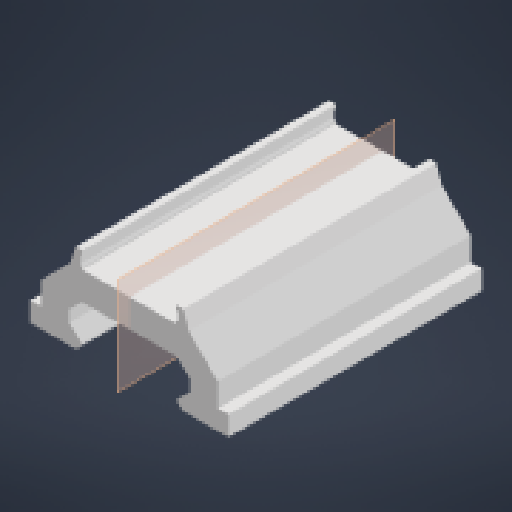
# Autodesk Inventor part: Rail clamp
Saved by Autodesk Inventor 2023 (Build 270158000, 158)
## iProperties
Created: 2023-10-16
Part Number: Rail clamp
Material: Generic
Document SubType Name: Modeling
Designer: nick_
Density: 1 g/cm^3
Appearance: Default
Author: nick_
Autodesk Inventor part; units mm, degrees
ref_plane "YZ Plane" through (0, 0, 0) normal (1, 0, 0) x (0, 1, 0)
ref_plane "XZ Plane" through (0, 0, 0) normal (0, 1, 0) x (-1, 0, 0)
ref_plane "XY Plane" through (0, 0, 0) normal (0, 0, 1) x (1, 0, 0)
sketch "Sketch1" plane through (0, 0, 0) normal (0, 0, 1) x (1, 0, 0)
  line L0 (6.1935, -6.1609) -> (-18.8065, -6.1609) construction
  line L1 (6.1935, -3.1609) -> (6.1935, -6.1609) construction
  line L2 (2.0882, -3.1609) -> (6.1935, -3.1609) construction
  line L3 (2.0882, -0.2145) -> (2.0882, -3.1609) construction
  line L4 (4.298, 1.9953) -> (2.0882, -0.2145) construction
  line L5 (4.298, 3.9511) -> (4.298, 1.9953) construction
  line L6 (2.0882, 6.1609) -> (4.298, 3.9511) construction
  line L7 (2.0882, 6.1609) -> (-14.7012, 6.1609) construction
  line L8 (-14.7012, 6.1609) -> (-16.911, 3.9511) construction
  line L9 (-16.911, 3.9511) -> (-16.911, 1.9953) construction
  line L10 (-16.911, 1.9953) -> (-14.7012, -0.2145) construction
  line L11 (-14.7012, -0.2145) -> (-14.7012, -3.1609) construction
  line L12 (-14.7012, -3.1609) -> (-18.8065, -3.1609) construction
  line L13 (-18.8065, -3.1609) -> (-18.8065, -6.1609) construction
  line L14 (2.1882, -3.0609) -> (6.2935, -3.0609)
  line L15 (6.2935, -3.0609) -> (6.2935, -6.2609)
  line L16 (6.2935, -6.2609) -> (-18.9065, -6.2609)
  line L17 (-18.9065, -6.2609) -> (-18.9065, -3.0609)
  line L18 (-18.9065, -3.0609) -> (-14.8012, -3.0609)
  line L19 (-14.8012, -3.0609) -> (-14.8012, -0.2559)
  line L20 (-14.8012, -0.2559) -> (-17.011, 1.9539)
  line L21 (-17.011, 1.9539) -> (-17.011, 3.9925)
  line L22 (-17.011, 3.9925) -> (-14.7427, 6.2609)
  line L23 (-14.7427, 6.2609) -> (2.1296, 6.2609)
  line L24 (2.1296, 6.2609) -> (4.398, 3.9925)
  line L25 (4.398, 3.9925) -> (4.398, 1.9539)
  line L26 (4.398, 1.9539) -> (2.1882, -0.2559)
  line L27 (2.1882, -0.2559) -> (2.1882, -3.0609)
  line L28 (11.2935, 1.9391) -> (9.398, 1.9391)
  line L29 (9.398, 1.9391) -> (9.398, 6.0636)
  line L30 (9.398, 6.0636) -> (4.2007, 11.2609)
  line L31 (4.2007, 11.2609) -> (-16.8137, 11.2609)
  line L32 (-16.8137, 11.2609) -> (-22.011, 6.0636)
  line L33 (-22.011, 6.0636) -> (-22.011, 1.9391)
  line L34 (-22.011, 1.9391) -> (-23.9065, 1.9391)
  line L35 (-23.9065, 1.9391) -> (-23.9065, -1.5609)
  line L36 (11.2935, -1.5609) -> (11.2935, 1.9391)
  line L37 (2.1882, -1.5609) -> (11.2935, -1.5609)
  line L38 (-14.8012, -1.5609) -> (-23.9065, -1.5609)
  point P0 (0, 0)
  point P1 (6.7408, -1.5609)
  point P2 (-19.3539, -1.5609)
  dimension "d0" = 0.1
  dimension "d1" = 5
  dimension "d2" = 1.5
  dimension "d3" = 5
  dimension "d5" = 5
  constraints: 50 end point, 2 midpoint, 2 perpendicular, 2 point on line, 1 horizontal alignment, 19 other
  measures "d0" distance between parallel lines of L3 L27
  measures "d1" distance between parallel lines of L36 L15
  measures "d2" distance between parallel lines of L37 L14
  measures "d3" distance between parallel lines of L31 L23
  measures "d5" distance between parallel lines of L35 L17
extrude "Extrusion1" add sketch "Sketch1" against normal blind 45 contours L27 L26 L25 L24 L23 L22 L21 L20 L19 L38 L35 L34 L33 L32 L31 L30 L29 L28 L36 L37
chamfer "Chamfer1" distance 1 angle 45 2 edges at (-14.8012, -1.5609, -22.5) (2.1882, -1.5609, -22.5)
sketch "Sketch3" plane through (0, 0, -45) normal (0, 0, -1) x (-1, 0, 0)
  line L0 (-2.2533, 11.7609) -> (14.8667, 11.7609) construction
  line L1 (14.8667, 11.7609) -> (14.8667, 13.2909) construction
  line L2 (-2.2533, 13.2909) -> (14.8667, 13.2909) construction
  line L3 (-2.2533, 11.7609) -> (-2.2533, 13.2909) construction
  line L4 (-2.1882, -0.5609) -> (-3.1882, -1.5609) construction
  line L5 (-2.1882, -0.5609) -> (-2.1882, -0.2559) construction
  line L6 (-2.1882, -0.2559) -> (-4.398, 1.9539) construction
  line L7 (-4.398, 1.9539) -> (-4.398, 3.9925) construction
  line L8 (-4.398, 3.9925) -> (-2.1296, 6.2609) construction
  line L9 (-2.1296, 6.2609) -> (14.7427, 6.2609) construction
  line L10 (14.7427, 6.2609) -> (17.011, 3.9925) construction
  line L11 (17.011, 3.9925) -> (17.011, 1.9539) construction
  line L12 (17.011, 1.9539) -> (14.8012, -0.2559) construction
  line L13 (14.8012, -0.2559) -> (14.8012, -0.5609) construction
  line L14 (15.8012, -1.5609) -> (14.8012, -0.5609) construction
  line L15 (15.8012, -1.5609) -> (23.9065, -1.5609) construction
  line L16 (23.9065, -1.5609) -> (23.9065, 1.9391) construction
  line L17 (23.9065, 1.9391) -> (22.011, 1.9391) construction
  line L18 (22.011, 1.9391) -> (22.011, 6.0636) construction
  line L19 (22.011, 6.0636) -> (16.8137, 11.2609) construction
  line L20 (16.8137, 11.2609) -> (-4.2007, 11.2609) construction
  line L21 (-4.2007, 11.2609) -> (-9.398, 6.0636) construction
  line L22 (-9.398, 6.0636) -> (-9.398, 1.9391) construction
  line L23 (-9.398, 1.9391) -> (-11.2935, 1.9391) construction
  line L24 (-11.2935, 1.9391) -> (-11.2935, -1.5609) construction
  line L25 (-11.2935, -1.5609) -> (-3.1882, -1.5609) construction
  line L26 (-2.0533, 11.2609) -> (-2.0533, 11.5609)
  line L27 (-2.0533, 11.5609) -> (-2.4533, 11.9609)
  line L28 (-2.4533, 11.9609) -> (-2.4533, 13.0909)
  line L29 (-2.4533, 13.0909) -> (-2.0533, 13.4909)
  line L30 (-2.0533, 13.4909) -> (-2.0533, 14.1683)
  line L31 (-2.0533, 14.1683) -> (-3.2638, 14.1683)
  line L32 (-3.2638, 14.1683) -> (-4.2007, 11.2609)
  line L33 (-4.2007, 11.2609) -> (-2.0533, 11.2609)
  line L34 (-2.2533, 13.2909) -> (-2.5848, 13.6224) construction
  line L35 (-2.2533, 13.2909) -> (-1.7845, 13.2909) construction
  point P0 (0, 0)
  point P1 (-2.2533, 13.2909)
  dimension "d15" = 0.2
  dimension "d16" = 135
  dimension "d17" = 0.2
  constraints: 20 end point, 4 point on line, 2 equal length, 2 midpoint, 2 perpendicular, 1 collinear, 1 horizontal, 1 parallel, 1 vertical
  measures "d15" distance between parallel lines of L3 L28
  measures "d16" angle of L35 L34
  measures "d17" distance from line of L2.start L30
extrude "Extrusion3" add sketch "Sketch3" against normal up to surface (45 mm away)
ref_plane "Work Plane1" through (-6.3065, -1.5609, 0) normal (1, 0, 0) x (0, 0, -1)
mirror "Mirror1" about plane through (-6.3065, -1.5609, 0) normal (1, 0, 0) of "Extrusion3"
sketch "Sketch4" plane through (2.0533, 11.2609, 0) normal (0, 1, 0) x (1, 0, 0)
  line L0 (-8.4373, 26.9134) -> (-8.4438, 26.9134) construction
  line L1 (-8.4438, 26.9134) -> (-8.4438, 27.0673) construction
  spline S0 degree 2 poles (-8.4438, 27.0673) (-8.3053, 27.184) (-7.9925, 27.3177) (-7.7834, 27.3177) knots 0 0 0 1 2 2 2 construction
  spline S1 degree 2 poles (-7.7834, 27.3177) (-7.5759, 27.3177) (-7.2615, 27.1848) (-7.1229, 27.0673) knots 0 0 0 1 2 2 2 construction
  line L2 (-7.1229, 27.0673) -> (-7.1229, 26.9134) construction
  line L3 (-7.1229, 26.9134) -> (-7.1294, 26.9134) construction
  spline S2 degree 2 poles (-7.1294, 26.9134) (-7.1756, 26.9652) (-7.3109, 27.0698) (-7.392, 27.1087) knots 0 0 0 1 2 2 2 construction
  spline S3 degree 2 poles (-7.392, 27.1087) (-7.4787, 27.1508) (-7.6715, 27.1994) (-7.7834, 27.1994) knots 0 0 0 1 2 2 2 construction
  spline S4 degree 2 poles (-7.7834, 27.1994) (-7.8944, 27.1994) (-8.0913, 27.15) (-8.1748, 27.1087) knots 0 0 0 1 2 2 2 construction
  spline S5 degree 2 poles (-8.1748, 27.1087) (-8.2583, 27.0682) (-8.3912, 26.9644) (-8.4373, 26.9134) knots 0 0 0 1 2 2 2 construction
  line L4 (-9.0457, 18.8862) -> (-10.0457, 18.8862) construction
  line L5 (-10.0457, 18.8862) -> (-10.0457, 19.1374) construction
  spline S6 degree 2 poles (-10.0457, 19.1374) (-10.0457, 19.2266) (-10.0166, 19.3514) (-9.9833, 19.3992) knots 0 0 0 1 2 2 2 construction
  spline S7 degree 2 poles (-9.9833, 19.3992) (-9.9452, 19.4551) (-9.8277, 19.5183) (-9.7443, 19.5183) knots 0 0 0 1 2 2 2 construction
  spline S8 degree 2 poles (-9.7443, 19.5183) (-9.6794, 19.5183) (-9.5628, 19.4721) (-9.5222, 19.4308) knots 0 0 0 1 2 2 2 construction
  spline S9 degree 2 poles (-9.5222, 19.4308) (-9.4712, 19.3789) (-9.4185, 19.2387) (-9.4185, 19.1318) knots 0 0 0 1 2 2 2 construction
  line L6 (-9.4185, 19.1318) -> (-9.4185, 19.0191) construction
  line L7 (-9.4185, 19.0191) -> (-9.0457, 19.0191) construction
  line L8 (-9.0457, 19.0191) -> (-9.0457, 18.8862) construction
  spline S10 degree 2 poles (-9.8205, 17.6472) (-9.7499, 17.6472) (-9.6381, 17.5726) (-9.6065, 17.507) knots 0 0 0 1 2 2 2 construction
  line L9 (-9.6065, 17.507) -> (-9.6017, 17.507) construction
  spline S11 degree 2 poles (-9.6017, 17.507) (-9.5773, 17.5961) (-9.4485, 17.6942) (-9.3529, 17.6942) knots 0 0 0 1 2 2 2 construction
  spline S12 degree 2 poles (-9.3529, 17.6942) (-9.2783, 17.6942) (-9.164, 17.6374) (-9.1268, 17.5904) knots 0 0 0 1 2 2 2 construction
  spline S13 degree 2 poles (-9.1268, 17.5904) (-9.083, 17.5337) (-9.0457, 17.4049) (-9.0457, 17.3028) knots 0 0 0 1 2 2 2 construction
  line L10 (-9.0457, 17.3028) -> (-9.0457, 17.0159) construction
  line L11 (-9.0457, 17.0159) -> (-10.0457, 17.0159) construction
  line L12 (-10.0457, 17.0159) -> (-10.0457, 17.2809) construction
  spline S14 degree 2 poles (-10.0457, 17.2809) (-10.0457, 17.3878) (-10.032, 17.4948) (-10.0052, 17.5434) knots 0 0 0 1 2 2 2 construction
  spline S15 degree 2 poles (-10.0052, 17.5434) (-9.9769, 17.5977) (-9.8837, 17.6472) (-9.8205, 17.6472) knots 0 0 0 1 2 2 2 construction
  spline S16 degree 2 poles (-10.066, 19.9195) (-10.066, 20.084) (-9.8067, 20.2387) (-9.5457, 20.2387) knots 0 0 0 1 2 2 2 construction
  spline S17 degree 2 poles (-9.5457, 20.2387) (-9.2767, 20.2387) (-9.0247, 20.0823) (-9.0247, 19.9195) knots 0 0 0 1 2 2 2 construction
  spline S18 degree 2 poles (-9.0247, 19.9195) (-9.0247, 19.7541) (-9.2816, 19.5994) (-9.5449, 19.5994) knots 0 0 0 1 2 2 2 construction
  spline S19 degree 2 poles (-9.5449, 19.5994) (-9.8156, 19.5994) (-10.066, 19.7558) (-10.066, 19.9195) knots 0 0 0 1 2 2 2 construction
  line L13 (-10.0457, 17.8263) -> (-10.0457, 18.0078) construction
  line L14 (-10.0457, 18.0078) -> (-9.489, 18.2574) construction
  line L15 (-9.489, 18.2574) -> (-10.0457, 18.4989) construction
  line L16 (-10.0457, 18.4989) -> (-10.0457, 18.6836) construction
  line L17 (-10.0457, 18.6836) -> (-9.0457, 18.6836) construction
  line L18 (-9.0457, 18.6836) -> (-9.0457, 18.5507) construction
  line L19 (-9.0457, 18.5507) -> (-9.9072, 18.5507) construction
  line L20 (-9.9072, 18.5507) -> (-9.3213, 18.2898) construction
  line L21 (-9.3213, 18.2898) -> (-9.3213, 18.2088) construction
  line L22 (-9.3213, 18.2088) -> (-9.9072, 17.9502) construction
  line L23 (-9.9072, 17.9502) -> (-9.0457, 17.9502) construction
  line L24 (-9.0457, 17.9502) -> (-9.0457, 17.8263) construction
  line L25 (-9.0457, 17.8263) -> (-10.0457, 17.8263) construction
  spline S20 degree 2 poles (-10.0684, 20.669) (-10.0684, 20.8052) (-9.9258, 20.9697) (-9.814, 20.9697) knots 0 0 0 1 2 2 2 construction
  spline S21 degree 2 poles (-9.814, 20.9697) (-9.7467, 20.9697) (-9.6154, 20.8911) (-9.5781, 20.8173) knots 0 0 0 1 2 2 2 construction
  line L26 (-9.5781, 20.8173) -> (-9.5741, 20.8173) construction
  spline S22 degree 2 poles (-9.5741, 20.8173) (-9.5336, 20.9049) (-9.4169, 20.9948) (-9.3245, 20.9948) knots 0 0 0 1 2 2 2 construction
  spline S23 degree 2 poles (-9.3245, 20.9948) (-9.1965, 20.9948) (-9.023, 20.8084) (-9.023, 20.669) knots 0 0 0 1 2 2 2 construction
  spline S24 degree 2 poles (-9.023, 20.669) (-9.023, 20.5945) (-9.0676, 20.4721) (-9.1089, 20.4292) knots 0 0 0 1 2 2 2 construction
  spline S25 degree 2 poles (-9.1089, 20.4292) (-9.1495, 20.387) (-9.2597, 20.3433) (-9.3221, 20.3433) knots 0 0 0 1 2 2 2 construction
  spline S26 degree 2 poles (-9.3221, 20.3433) (-9.4031, 20.3433) (-9.5393, 20.43) (-9.5798, 20.5126) knots 0 0 0 1 2 2 2 construction
  line L27 (-9.5798, 20.5126) -> (-9.5838, 20.5126) construction
  spline S27 degree 2 poles (-9.5838, 20.5126) (-9.6268, 20.4389) (-9.7289, 20.3676) (-9.8051, 20.3676) knots 0 0 0 1 2 2 2 construction
  spline S28 degree 2 poles (-9.8051, 20.3676) (-9.9177, 20.3676) (-10.0684, 20.5378) (-10.0684, 20.669) knots 0 0 0 1 2 2 2 construction
  line L28 (-9.5303, 21.169) -> (-10.0457, 21.169) construction
  line L29 (-10.0457, 21.169) -> (-10.0457, 21.7177) construction
  line L30 (-10.0457, 21.7177) -> (-9.9282, 21.7177) construction
  line L31 (-9.9282, 21.7177) -> (-9.9282, 21.2979) construction
  line L32 (-9.9282, 21.2979) -> (-9.6616, 21.2979) construction
  spline S29 degree 2 poles (-9.6616, 21.2979) (-9.6649, 21.3222) (-9.6673, 21.3692) (-9.6673, 21.3887) knots 0 0 0 1 2 2 2 construction
  spline S30 degree 2 poles (-9.6673, 21.3887) (-9.6673, 21.4656) (-9.6422, 21.5718) (-9.6049, 21.6204) knots 0 0 0 1 2 2 2 construction
  spline S31 degree 2 poles (-9.6049, 21.6204) (-9.5676, 21.6699) (-9.4542, 21.7233) (-9.3634, 21.7233) knots 0 0 0 1 2 2 2 construction
  spline S32 degree 2 poles (-9.3634, 21.7233) (-9.2913, 21.7233) (-9.1681, 21.6771) (-9.1227, 21.635) knots 0 0 0 1 2 2 2 construction
  spline S33 degree 2 poles (-9.1227, 21.635) (-9.0773, 21.5929) (-9.0247, 21.4673) (-9.0247, 21.3895) knots 0 0 0 1 2 2 2 construction
  spline S34 degree 2 poles (-9.0247, 21.3895) (-9.0247, 21.3182) (-9.0563, 21.1788) (-9.0814, 21.1277) knots 0 0 0 1 2 2 2 construction
  line L33 (-9.0814, 21.1277) -> (-9.2232, 21.1277) construction
  line L34 (-9.2232, 21.1277) -> (-9.2232, 21.1374) construction
  spline S35 degree 2 poles (-9.2232, 21.1374) (-9.2119, 21.1528) (-9.1827, 21.2104) (-9.1697, 21.2452) knots 0 0 0 1 2 2 2 construction
  spline S36 degree 2 poles (-9.1697, 21.2452) (-9.1559, 21.2849) (-9.1405, 21.3506) (-9.1405, 21.3919) knots 0 0 0 1 2 2 2 construction
  spline S37 degree 2 poles (-9.1405, 21.3919) (-9.1405, 21.4324) (-9.1697, 21.5086) (-9.2013, 21.5361) knots 0 0 0 1 2 2 2 construction
  spline S38 degree 2 poles (-9.2013, 21.5361) (-9.2313, 21.5613) (-9.3107, 21.5872) (-9.3642, 21.5872) knots 0 0 0 1 2 2 2 construction
  spline S39 degree 2 poles (-9.3642, 21.5872) (-9.4177, 21.5872) (-9.4858, 21.558) (-9.5085, 21.5305) knots 0 0 0 1 2 2 2 construction
  spline S40 degree 2 poles (-9.5085, 21.5305) (-9.5336, 21.5021) (-9.5546, 21.4178) (-9.5546, 21.3668) knots 0 0 0 1 2 2 2 construction
  spline S41 degree 2 poles (-9.5546, 21.3668) (-9.5546, 21.3117) (-9.5376, 21.2023) (-9.5303, 21.169) knots 0 0 0 1 2 2 2 construction
  spline S42 degree 2 poles (-8.1748, 12.0301) (-8.0921, 11.9895) (-7.8936, 11.9393) (-7.7834, 11.9393) knots 0 0 0 1 2 2 2 construction
  spline S43 degree 2 poles (-7.7834, 11.9393) (-7.6683, 11.9393) (-7.4779, 11.9879) (-7.392, 12.0301) knots 0 0 0 1 2 2 2 construction
  spline S44 degree 2 poles (-7.392, 12.0301) (-7.3093, 12.0706) (-7.1756, 12.1735) (-7.1294, 12.2254) knots 0 0 0 1 2 2 2 construction
  line L35 (-7.1294, 12.2254) -> (-7.1229, 12.2254) construction
  line L36 (-7.1229, 12.2254) -> (-7.1229, 12.0714) construction
  spline S45 degree 2 poles (-7.1229, 12.0714) (-7.2615, 11.9547) (-7.5719, 11.821) (-7.7834, 11.821) knots 0 0 0 1 2 2 2 construction
  spline S46 degree 2 poles (-7.7834, 11.821) (-7.99, 11.821) (-8.3053, 11.9531) (-8.4438, 12.0714) knots 0 0 0 1 2 2 2 construction
  line L37 (-8.4438, 12.0714) -> (-8.4438, 12.2254) construction
  line L38 (-8.4438, 12.2254) -> (-8.4373, 12.2254) construction
  spline S47 degree 2 poles (-8.4373, 12.2254) (-8.3879, 12.1711) (-8.2599, 12.0722) (-8.1748, 12.0301) knots 0 0 0 1 2 2 2 construction
  line L39 (-8.2972, 12.7254) -> (-8.2972, 12.5981) construction
  line L40 (-8.2972, 12.5981) -> (-7.5014, 12.5981) construction
  line L41 (-7.5014, 12.5981) -> (-7.5014, 12.7254) construction
  line L42 (-7.5014, 12.7254) -> (-7.3993, 12.7254) construction
  line L43 (-7.3993, 12.7254) -> (-7.3993, 12.338) construction
  line L44 (-7.3993, 12.338) -> (-7.5014, 12.338) construction
  line L45 (-7.5014, 12.338) -> (-7.5014, 12.4652) construction
  line L46 (-7.5014, 12.4652) -> (-8.2972, 12.4652) construction
  line L47 (-8.2972, 12.4652) -> (-8.2972, 12.338) construction
  line L48 (-8.2972, 12.338) -> (-8.3993, 12.338) construction
  line L49 (-8.3993, 12.338) -> (-8.3993, 12.7254) construction
  line L50 (-8.3993, 12.7254) -> (-8.2972, 12.7254) construction
  line L51 (-8.2809, 13.5917) -> (-8.2809, 13.2562) construction
  line L52 (-8.2809, 13.2562) -> (-7.3993, 13.2562) construction
  line L53 (-7.3993, 13.2562) -> (-7.3993, 13.1233) construction
  line L54 (-7.3993, 13.1233) -> (-8.2809, 13.1233) construction
  line L55 (-8.2809, 13.1233) -> (-8.2809, 12.7878) construction
  line L56 (-8.2809, 12.7878) -> (-8.3993, 12.7878) construction
  line L57 (-8.3993, 12.7878) -> (-8.3993, 13.5917) construction
  line L58 (-8.3993, 13.5917) -> (-8.2809, 13.5917) construction
  spline S48 degree 2 poles (-7.601, 13.8664) (-7.5492, 13.9093) (-7.4949, 14.0309) (-7.4949, 14.1071) knots 0 0 0 1 2 2 2 construction
  spline S49 degree 2 poles (-7.4949, 14.1071) (-7.4949, 14.163) (-7.5111, 14.2748) (-7.5273, 14.3129) knots 0 0 0 1 2 2 2 construction
  line L59 (-7.5273, 14.3129) -> (-7.7858, 14.3129) construction
  line L60 (-7.7858, 14.3129) -> (-7.7858, 14.0811) construction
  line L61 (-7.7858, 14.0811) -> (-7.9025, 14.0811) construction
  line L62 (-7.9025, 14.0811) -> (-7.9025, 14.4442) construction
  line L63 (-7.9025, 14.4442) -> (-7.4657, 14.4442) construction
  spline S50 degree 2 poles (-7.4657, 14.4442) (-7.4544, 14.419) (-7.4195, 14.3331) (-7.409, 14.2967) knots 0 0 0 1 2 2 2 construction
  spline S51 degree 2 poles (-7.409, 14.2967) (-7.3944, 14.2472) (-7.3798, 14.1678) (-7.3798, 14.1119) knots 0 0 0 1 2 2 2 construction
  spline S52 degree 2 poles (-7.3798, 14.1119) (-7.3798, 14.0058) (-7.4446, 13.8299) (-7.5103, 13.7667) knots 0 0 0 1 2 2 2 construction
  spline S53 degree 2 poles (-7.5103, 13.7667) (-7.5767, 13.7035) (-7.7728, 13.6362) (-7.9001, 13.6362) knots 0 0 0 1 2 2 2 construction
  spline S54 degree 2 poles (-7.9001, 13.6362) (-8.0208, 13.6362) (-8.2121, 13.7043) (-8.2801, 13.7675) knots 0 0 0 1 2 2 2 construction
  spline S55 degree 2 poles (-8.2801, 13.7675) (-8.3458, 13.8283) (-8.4171, 14.0066) (-8.4171, 14.1127) knots 0 0 0 1 2 2 2 construction
  spline S56 degree 2 poles (-8.4171, 14.1127) (-8.4171, 14.1638) (-8.4025, 14.2562) (-8.3895, 14.2983) knots 0 0 0 1 2 2 2 construction
  spline S57 degree 2 poles (-8.3895, 14.2983) (-8.3798, 14.3323) (-8.3442, 14.415) (-8.3312, 14.4401) knots 0 0 0 1 2 2 2 construction
  line L64 (-8.3312, 14.4401) -> (-8.1707, 14.4401) construction
  line L65 (-8.1707, 14.4401) -> (-8.1707, 14.4288) construction
  spline S58 degree 2 poles (-8.1707, 14.4288) (-8.1926, 14.4036) (-8.2323, 14.351) (-8.255, 14.3024) knots 0 0 0 1 2 2 2 construction
  spline S59 degree 2 poles (-8.255, 14.3024) (-8.2753, 14.2618) (-8.302, 14.1573) (-8.302, 14.0973) knots 0 0 0 1 2 2 2 construction
  spline S60 degree 2 poles (-8.302, 14.0973) (-8.302, 13.9531) (-8.0848, 13.7748) (-7.9041, 13.7748) knots 0 0 0 1 2 2 2 construction
  spline S61 degree 2 poles (-7.9041, 13.7748) (-7.8036, 13.7748) (-7.6529, 13.8218) (-7.601, 13.8664) knots 0 0 0 1 2 2 2 construction
  line L66 (-7.4398, 14.5746) -> (-7.5816, 14.5746) construction
  line L67 (-7.5816, 14.5746) -> (-7.5816, 14.5844) construction
  spline S62 degree 2 poles (-7.5816, 14.5844) (-7.5508, 14.6265) (-7.4941, 14.7691) (-7.4941, 14.8396) knots 0 0 0 1 2 2 2 construction
  spline S63 degree 2 poles (-7.4941, 14.8396) (-7.4941, 14.881) (-7.52, 14.9636) (-7.55, 14.9912) knots 0 0 0 1 2 2 2 construction
  spline S64 degree 2 poles (-7.55, 14.9912) (-7.58, 15.0179) (-7.6513, 15.0463) (-7.7056, 15.0463) knots 0 0 0 1 2 2 2 construction
  spline S65 degree 2 poles (-7.7056, 15.0463) (-7.7599, 15.0463) (-7.8304, 15.0147) (-7.8506, 14.9863) knots 0 0 0 1 2 2 2 construction
  spline S66 degree 2 poles (-7.8506, 14.9863) (-7.8709, 14.9579) (-7.8863, 14.881) (-7.8863, 14.8356) knots 0 0 0 1 2 2 2 construction
  line L68 (-7.8863, 14.8356) -> (-7.8863, 14.7789) construction
  line L69 (-7.8863, 14.7789) -> (-7.9973, 14.7789) construction
  line L70 (-7.9973, 14.7789) -> (-7.9973, 14.8234) construction
  spline S67 degree 2 poles (-7.9973, 14.8234) (-7.9973, 14.9134) (-8.0832, 15.0268) (-8.1651, 15.0268) knots 0 0 0 1 2 2 2 construction
  spline S68 degree 2 poles (-8.1651, 15.0268) (-8.2032, 15.0268) (-8.2574, 14.9977) (-8.2737, 14.9742) knots 0 0 0 1 2 2 2 construction
  spline S69 degree 2 poles (-8.2737, 14.9742) (-8.2907, 14.949) (-8.3044, 14.8874) (-8.3044, 14.8526) knots 0 0 0 1 2 2 2 construction
  spline S70 degree 2 poles (-8.3044, 14.8526) (-8.3044, 14.8161) (-8.2866, 14.744) (-8.2728, 14.7092) knots 0 0 0 1 2 2 2 construction
  spline S71 degree 2 poles (-8.2728, 14.7092) (-8.2591, 14.6767) (-8.2299, 14.6289) (-8.2169, 14.6103) knots 0 0 0 1 2 2 2 construction
  line L71 (-8.2169, 14.6103) -> (-8.2169, 14.6022) construction
  line L72 (-8.2169, 14.6022) -> (-8.3587, 14.6022) construction
  spline S72 degree 2 poles (-8.3587, 14.6022) (-8.3822, 14.646) (-8.4203, 14.7959) (-8.4203, 14.8631) knots 0 0 0 1 2 2 2 construction
  spline S73 degree 2 poles (-8.4203, 14.8631) (-8.4203, 14.9312) (-8.3928, 15.0325) (-8.3636, 15.0738) knots 0 0 0 1 2 2 2 construction
  spline S74 degree 2 poles (-8.3636, 15.0738) (-8.332, 15.1176) (-8.2404, 15.163) (-8.1788, 15.163) knots 0 0 0 1 2 2 2 construction
  spline S75 degree 2 poles (-8.1788, 15.163) (-8.0962, 15.163) (-7.9714, 15.0544) (-7.9552, 14.9782) knots 0 0 0 1 2 2 2 construction
  line L73 (-7.9552, 14.9782) -> (-7.9455, 14.9782) construction
  spline S76 degree 2 poles (-7.9455, 14.9782) (-7.939, 15.0098) (-7.9098, 15.0819) (-7.8806, 15.1127) knots 0 0 0 1 2 2 2 construction
  spline S77 degree 2 poles (-7.8806, 15.1127) (-7.8523, 15.1435) (-7.7615, 15.1824) (-7.6959, 15.1824) knots 0 0 0 1 2 2 2 construction
  spline S78 degree 2 poles (-7.6959, 15.1824) (-7.6286, 15.1824) (-7.5143, 15.1362) (-7.4706, 15.0941) knots 0 0 0 1 2 2 2 construction
  spline S79 degree 2 poles (-7.4706, 15.0941) (-7.4252, 15.0503) (-7.3782, 14.9263) (-7.3782, 14.8477) knots 0 0 0 1 2 2 2 construction
  spline S80 degree 2 poles (-7.3782, 14.8477) (-7.3782, 14.7724) (-7.4147, 14.6249) (-7.4398, 14.5746) knots 0 0 0 1 2 2 2 construction
  spline S81 degree 2 poles (-8.3604, 15.3542) (-8.3806, 15.3955) (-8.4203, 15.5438) (-8.4203, 15.6103) knots 0 0 0 1 2 2 2 construction
  spline S82 degree 2 poles (-8.4203, 15.6103) (-8.4203, 15.7505) (-8.272, 15.9085) (-8.1456, 15.9085) knots 0 0 0 1 2 2 2 construction
  spline S83 degree 2 poles (-8.1456, 15.9085) (-8.0865, 15.9085) (-7.9876, 15.881) (-7.9455, 15.8566) knots 0 0 0 1 2 2 2 construction
  spline S84 degree 2 poles (-7.9455, 15.8566) (-7.9017, 15.8323) (-7.8158, 15.7618) (-7.7745, 15.7229) knots 0 0 0 1 2 2 2 construction
  spline S85 degree 2 poles (-7.7745, 15.7229) (-7.7056, 15.6597) (-7.5581, 15.5049) (-7.5151, 15.4588) knots 0 0 0 1 2 2 2 construction
  line L74 (-7.5151, 15.4588) -> (-7.5151, 15.9498) construction
  line L75 (-7.5151, 15.9498) -> (-7.3993, 15.9498) construction
  line L76 (-7.3993, 15.9498) -> (-7.3993, 15.3331) construction
  line L77 (-7.3993, 15.3331) -> (-7.5411, 15.3331) construction
  spline S86 degree 2 poles (-7.5411, 15.3331) (-7.6035, 15.3996) (-7.7194, 15.5179) (-7.7818, 15.5746) knots 0 0 0 1 2 2 2 construction
  spline S87 degree 2 poles (-7.7818, 15.5746) (-7.9074, 15.6889) (-8.0581, 15.7724) (-8.1383, 15.7724) knots 0 0 0 1 2 2 2 construction
  spline S88 degree 2 poles (-8.1383, 15.7724) (-8.1805, 15.7724) (-8.2437, 15.7464) (-8.2639, 15.7229) knots 0 0 0 1 2 2 2 construction
  spline S89 degree 2 poles (-8.2639, 15.7229) (-8.2842, 15.6994) (-8.3044, 15.6378) (-8.3044, 15.6006) knots 0 0 0 1 2 2 2 construction
  spline S90 degree 2 poles (-8.3044, 15.6006) (-8.3044, 15.5649) (-8.2866, 15.492) (-8.2728, 15.4588) knots 0 0 0 1 2 2 2 construction
  spline S91 degree 2 poles (-8.2728, 15.4588) (-8.2615, 15.4304) (-8.2291, 15.3777) (-8.2177, 15.3615) knots 0 0 0 1 2 2 2 construction
  line L78 (-8.2177, 15.3615) -> (-8.2177, 15.3542) construction
  line L79 (-8.2177, 15.3542) -> (-8.3604, 15.3542) construction
  spline S92 degree 2 poles (-8.4195, 16.3866) (-8.4195, 16.5511) (-8.1602, 16.7059) (-7.8993, 16.7059) knots 0 0 0 1 2 2 2 construction
  spline S93 degree 2 poles (-7.8993, 16.7059) (-7.6302, 16.7059) (-7.3782, 16.5495) (-7.3782, 16.3866) knots 0 0 0 1 2 2 2 construction
  spline S94 degree 2 poles (-7.3782, 16.3866) (-7.3782, 16.2213) (-7.6351, 16.0665) (-7.8985, 16.0665) knots 0 0 0 1 2 2 2 construction
  spline S95 degree 2 poles (-7.8985, 16.0665) (-8.1691, 16.0665) (-8.4195, 16.2229) (-8.4195, 16.3866) knots 0 0 0 1 2 2 2 construction
  line L80 (-7.6788, 18.1597) -> (-7.3993, 18.069) construction
  line L81 (-7.3993, 18.069) -> (-7.3993, 17.9344) construction
  line L82 (-7.3993, 17.9344) -> (-8.3993, 18.2716) construction
  line L83 (-8.3993, 18.2716) -> (-8.3993, 18.4353) construction
  line L84 (-8.3993, 18.4353) -> (-7.3993, 18.7724) construction
  line L85 (-7.3993, 18.7724) -> (-7.3993, 18.6322) construction
  line L86 (-7.3993, 18.6322) -> (-7.6788, 18.5414) construction
  line L87 (-7.6788, 18.5414) -> (-7.6788, 18.1597) construction
  spline S96 degree 2 poles (-7.9082, 17.0836) (-7.9082, 17.0284) (-7.8912, 16.919) (-7.8839, 16.8858) knots 0 0 0 1 2 2 2 construction
  line L88 (-7.8839, 16.8858) -> (-8.3993, 16.8858) construction
  line L89 (-8.3993, 16.8858) -> (-8.3993, 17.4344) construction
  line L90 (-8.3993, 17.4344) -> (-8.2818, 17.4344) construction
  line L91 (-8.2818, 17.4344) -> (-8.2818, 17.0147) construction
  line L92 (-8.2818, 17.0147) -> (-8.0151, 17.0147) construction
  spline S97 degree 2 poles (-8.0151, 17.0147) (-8.0184, 17.039) (-8.0208, 17.086) (-8.0208, 17.1054) knots 0 0 0 1 2 2 2 construction
  spline S98 degree 2 poles (-8.0208, 17.1054) (-8.0208, 17.1824) (-7.9957, 17.2886) (-7.9584, 17.3372) knots 0 0 0 1 2 2 2 construction
  spline S99 degree 2 poles (-7.9584, 17.3372) (-7.9211, 17.3866) (-7.8077, 17.4401) (-7.7169, 17.4401) knots 0 0 0 1 2 2 2 construction
  spline S100 degree 2 poles (-7.7169, 17.4401) (-7.6448, 17.4401) (-7.5216, 17.3939) (-7.4762, 17.3518) knots 0 0 0 1 2 2 2 construction
  spline S101 degree 2 poles (-7.4762, 17.3518) (-7.4309, 17.3096) (-7.3782, 17.184) (-7.3782, 17.1062) knots 0 0 0 1 2 2 2 construction
  spline S102 degree 2 poles (-7.3782, 17.1062) (-7.3782, 17.0349) (-7.4098, 16.8955) (-7.4349, 16.8445) knots 0 0 0 1 2 2 2 construction
  line L93 (-7.4349, 16.8445) -> (-7.5767, 16.8445) construction
  line L94 (-7.5767, 16.8445) -> (-7.5767, 16.8542) construction
  spline S103 degree 2 poles (-7.5767, 16.8542) (-7.5654, 16.8696) (-7.5362, 16.9271) (-7.5232, 16.962) knots 0 0 0 1 2 2 2 construction
  spline S104 degree 2 poles (-7.5232, 16.962) (-7.5095, 17.0017) (-7.4941, 17.0673) (-7.4941, 17.1087) knots 0 0 0 1 2 2 2 construction
  spline S105 degree 2 poles (-7.4941, 17.1087) (-7.4941, 17.1492) (-7.5232, 17.2254) (-7.5549, 17.2529) knots 0 0 0 1 2 2 2 construction
  spline S106 degree 2 poles (-7.5549, 17.2529) (-7.5848, 17.278) (-7.6643, 17.304) (-7.7177, 17.304) knots 0 0 0 1 2 2 2 construction
  spline S107 degree 2 poles (-7.7177, 17.304) (-7.7712, 17.304) (-7.8393, 17.2748) (-7.862, 17.2472) knots 0 0 0 1 2 2 2 construction
  spline S108 degree 2 poles (-7.862, 17.2472) (-7.8871, 17.2189) (-7.9082, 17.1346) (-7.9082, 17.0836) knots 0 0 0 1 2 2 2 construction
  spline S109 degree 2 poles (-8.3993, 19.0949) (-8.3993, 19.2359) (-8.3571, 19.3964) (-8.3198, 19.4531) knots 0 0 0 1 2 2 2 construction
  spline S110 degree 2 poles (-8.3198, 19.4531) (-8.2558, 19.5495) (-8.0443, 19.6557) (-7.8985, 19.6557) knots 0 0 0 1 2 2 2 construction
  spline S111 degree 2 poles (-7.8985, 19.6557) (-7.7615, 19.6557) (-7.5411, 19.5447) (-7.4795, 19.4515) knots 0 0 0 1 2 2 2 construction
  spline S112 degree 2 poles (-7.4795, 19.4515) (-7.4317, 19.3753) (-7.3993, 19.2189) (-7.3993, 19.0973) knots 0 0 0 1 2 2 2 construction
  line L95 (-7.3993, 19.0973) -> (-7.3993, 18.8672) construction
  line L96 (-7.3993, 18.8672) -> (-8.3993, 18.8672) construction
  line L97 (-8.3993, 18.8672) -> (-8.3993, 19.0949) construction
  line L98 (-7.5176, 20.731) -> (-7.5176, 21.1776) construction
  line L99 (-7.5176, 21.1776) -> (-7.3993, 21.1776) construction
  line L100 (-7.3993, 21.1776) -> (-7.3993, 20.5981) construction
  line L101 (-7.3993, 20.5981) -> (-8.3993, 20.5981) construction
  line L102 (-8.3993, 20.5981) -> (-8.3993, 20.731) construction
  line L103 (-8.3993, 20.731) -> (-7.5176, 20.731) construction
  line L104 (-8.0079, 20.1046) -> (-8.3993, 20.3477) construction
  line L105 (-8.3993, 20.3477) -> (-8.3993, 20.4912) construction
  line L106 (-8.3993, 20.4912) -> (-7.9066, 20.1784) construction
  line L107 (-7.9066, 20.1784) -> (-7.3993, 20.4912) construction
  line L108 (-7.3993, 20.4912) -> (-7.3993, 20.3388) construction
  line L109 (-7.3993, 20.3388) -> (-7.798, 20.0957) construction
  line L110 (-7.798, 20.0957) -> (-7.3993, 19.8477) construction
  line L111 (-7.3993, 19.8477) -> (-7.3993, 19.7043) construction
  line L112 (-7.3993, 19.7043) -> (-7.9001, 20.0228) construction
  line L113 (-7.9001, 20.0228) -> (-8.3993, 19.714) construction
  line L114 (-8.3993, 19.714) -> (-8.3993, 19.8664) construction
  line L115 (-8.3993, 19.8664) -> (-8.0079, 20.1046) construction
  line L116 (-7.8839, 21.9579) -> (-8.3993, 22.4053) construction
  line L117 (-8.3993, 22.4053) -> (-8.3993, 22.5284) construction
  line L118 (-8.3993, 22.5284) -> (-7.8506, 22.5284) construction
  line L119 (-7.8506, 22.5284) -> (-7.8506, 22.6476) construction
  line L120 (-7.8506, 22.6476) -> (-7.7429, 22.6476) construction
  line L121 (-7.7429, 22.6476) -> (-7.7429, 22.5284) construction
  line L122 (-7.7429, 22.5284) -> (-7.3993, 22.5284) construction
  line L123 (-7.3993, 22.5284) -> (-7.3993, 22.3996) construction
  line L124 (-7.3993, 22.3996) -> (-7.7429, 22.3996) construction
  line L125 (-7.7429, 22.3996) -> (-7.7429, 21.9579) construction
  line L126 (-7.7429, 21.9579) -> (-7.8839, 21.9579) construction
  line L127 (-7.5816, 21.2456) -> (-7.5816, 21.2554) construction
  spline S113 degree 2 poles (-7.5816, 21.2554) (-7.5508, 21.2975) (-7.4941, 21.4401) (-7.4941, 21.5106) knots 0 0 0 1 2 2 2 construction
  spline S114 degree 2 poles (-7.4941, 21.5106) (-7.4941, 21.5519) (-7.52, 21.6346) (-7.55, 21.6622) knots 0 0 0 1 2 2 2 construction
  spline S115 degree 2 poles (-7.55, 21.6622) (-7.58, 21.6889) (-7.6513, 21.7173) (-7.7056, 21.7173) knots 0 0 0 1 2 2 2 construction
  spline S116 degree 2 poles (-7.7056, 21.7173) (-7.7599, 21.7173) (-7.8304, 21.6857) (-7.8506, 21.6573) knots 0 0 0 1 2 2 2 construction
  spline S117 degree 2 poles (-7.8506, 21.6573) (-7.8709, 21.6289) (-7.8863, 21.5519) (-7.8863, 21.5066) knots 0 0 0 1 2 2 2 construction
  line L128 (-7.8863, 21.5066) -> (-7.8863, 21.4498) construction
  line L129 (-7.8863, 21.4498) -> (-7.9973, 21.4498) construction
  line L130 (-7.9973, 21.4498) -> (-7.9973, 21.4944) construction
  spline S118 degree 2 poles (-7.9973, 21.4944) (-7.9973, 21.5844) (-8.0832, 21.6978) (-8.1651, 21.6978) knots 0 0 0 1 2 2 2 construction
  spline S119 degree 2 poles (-8.1651, 21.6978) (-8.2032, 21.6978) (-8.2574, 21.6686) (-8.2737, 21.6451) knots 0 0 0 1 2 2 2 construction
  spline S120 degree 2 poles (-8.2737, 21.6451) (-8.2907, 21.62) (-8.3044, 21.5584) (-8.3044, 21.5236) knots 0 0 0 1 2 2 2 construction
  spline S121 degree 2 poles (-8.3044, 21.5236) (-8.3044, 21.4871) (-8.2866, 21.415) (-8.2728, 21.3801) knots 0 0 0 1 2 2 2 construction
  spline S122 degree 2 poles (-8.2728, 21.3801) (-8.2591, 21.3477) (-8.2299, 21.2999) (-8.2169, 21.2813) knots 0 0 0 1 2 2 2 construction
  line L131 (-8.2169, 21.2813) -> (-8.2169, 21.2732) construction
  line L132 (-8.2169, 21.2732) -> (-8.3587, 21.2732) construction
  spline S123 degree 2 poles (-8.3587, 21.2732) (-8.3822, 21.3169) (-8.4203, 21.4669) (-8.4203, 21.5341) knots 0 0 0 1 2 2 2 construction
  spline S124 degree 2 poles (-8.4203, 21.5341) (-8.4203, 21.6022) (-8.3928, 21.7035) (-8.3636, 21.7448) knots 0 0 0 1 2 2 2 construction
  spline S125 degree 2 poles (-8.3636, 21.7448) (-8.332, 21.7886) (-8.2404, 21.834) (-8.1788, 21.834) knots 0 0 0 1 2 2 2 construction
  spline S126 degree 2 poles (-8.1788, 21.834) (-8.0962, 21.834) (-7.9714, 21.7254) (-7.9552, 21.6492) knots 0 0 0 1 2 2 2 construction
  line L133 (-7.9552, 21.6492) -> (-7.9455, 21.6492) construction
  spline S127 degree 2 poles (-7.9455, 21.6492) (-7.939, 21.6808) (-7.9098, 21.7529) (-7.8806, 21.7837) knots 0 0 0 1 2 2 2 construction
  spline S128 degree 2 poles (-7.8806, 21.7837) (-7.8523, 21.8145) (-7.7615, 21.8534) (-7.6959, 21.8534) knots 0 0 0 1 2 2 2 construction
  spline S129 degree 2 poles (-7.6959, 21.8534) (-7.6286, 21.8534) (-7.5143, 21.8072) (-7.4706, 21.7651) knots 0 0 0 1 2 2 2 construction
  spline S130 degree 2 poles (-7.4706, 21.7651) (-7.4252, 21.7213) (-7.3782, 21.5973) (-7.3782, 21.5187) knots 0 0 0 1 2 2 2 construction
  spline S131 degree 2 poles (-7.3782, 21.5187) (-7.3782, 21.4434) (-7.4147, 21.2959) (-7.4398, 21.2456) knots 0 0 0 1 2 2 2 construction
  line L134 (-7.4398, 21.2456) -> (-7.5816, 21.2456) construction
  spline S132 degree 2 poles (-7.9082, 23.0041) (-7.9082, 22.949) (-7.8912, 22.8396) (-7.8839, 22.8064) knots 0 0 0 1 2 2 2 construction
  line L135 (-7.8839, 22.8064) -> (-8.3993, 22.8064) construction
  line L136 (-8.3993, 22.8064) -> (-8.3993, 23.355) construction
  line L137 (-8.3993, 23.355) -> (-8.2818, 23.355) construction
  line L138 (-8.2818, 23.355) -> (-8.2818, 22.9353) construction
  line L139 (-8.2818, 22.9353) -> (-8.0151, 22.9353) construction
  spline S133 degree 2 poles (-8.0151, 22.9353) (-8.0184, 22.9596) (-8.0208, 23.0066) (-8.0208, 23.026) knots 0 0 0 1 2 2 2 construction
  spline S134 degree 2 poles (-8.0208, 23.026) (-8.0208, 23.103) (-7.9957, 23.2092) (-7.9584, 23.2578) knots 0 0 0 1 2 2 2 construction
  spline S135 degree 2 poles (-7.9584, 23.2578) (-7.9211, 23.3072) (-7.8077, 23.3607) (-7.7169, 23.3607) knots 0 0 0 1 2 2 2 construction
  spline S136 degree 2 poles (-7.7169, 23.3607) (-7.6448, 23.3607) (-7.5216, 23.3145) (-7.4762, 23.2724) knots 0 0 0 1 2 2 2 construction
  spline S137 degree 2 poles (-7.4762, 23.2724) (-7.4309, 23.2302) (-7.3782, 23.1046) (-7.3782, 23.0268) knots 0 0 0 1 2 2 2 construction
  spline S138 degree 2 poles (-7.3782, 23.0268) (-7.3782, 22.9555) (-7.4098, 22.8161) (-7.4349, 22.7651) knots 0 0 0 1 2 2 2 construction
  line L140 (-7.4349, 22.7651) -> (-7.5767, 22.7651) construction
  line L141 (-7.5767, 22.7651) -> (-7.5767, 22.7748) construction
  spline S139 degree 2 poles (-7.5767, 22.7748) (-7.5654, 22.7902) (-7.5362, 22.8477) (-7.5232, 22.8826) knots 0 0 0 1 2 2 2 construction
  spline S140 degree 2 poles (-7.5232, 22.8826) (-7.5095, 22.9223) (-7.4941, 22.9879) (-7.4941, 23.0293) knots 0 0 0 1 2 2 2 construction
  spline S141 degree 2 poles (-7.4941, 23.0293) (-7.4941, 23.0698) (-7.5232, 23.146) (-7.5549, 23.1735) knots 0 0 0 1 2 2 2 construction
  spline S142 degree 2 poles (-7.5549, 23.1735) (-7.5848, 23.1986) (-7.6643, 23.2246) (-7.7177, 23.2246) knots 0 0 0 1 2 2 2 construction
  spline S143 degree 2 poles (-7.7177, 23.2246) (-7.7712, 23.2246) (-7.8393, 23.1954) (-7.862, 23.1678) knots 0 0 0 1 2 2 2 construction
  spline S144 degree 2 poles (-7.862, 23.1678) (-7.8871, 23.1395) (-7.9082, 23.0552) (-7.9082, 23.0041) knots 0 0 0 1 2 2 2 construction
  line L142 (-7.8839, 23.9863) -> (-8.3993, 23.9863) construction
  line L143 (-8.3993, 23.9863) -> (-8.3993, 24.5349) construction
  line L144 (-8.3993, 24.5349) -> (-8.2818, 24.5349) construction
  line L145 (-8.2818, 24.5349) -> (-8.2818, 24.1152) construction
  line L146 (-8.2818, 24.1152) -> (-8.0151, 24.1152) construction
  spline S145 degree 2 poles (-8.0151, 24.1152) (-8.0184, 24.1395) (-8.0208, 24.1865) (-8.0208, 24.2059) knots 0 0 0 1 2 2 2 construction
  spline S146 degree 2 poles (-8.0208, 24.2059) (-8.0208, 24.2829) (-7.9957, 24.3891) (-7.9584, 24.4377) knots 0 0 0 1 2 2 2 construction
  spline S147 degree 2 poles (-7.9584, 24.4377) (-7.9211, 24.4871) (-7.8077, 24.5406) (-7.7169, 24.5406) knots 0 0 0 1 2 2 2 construction
  spline S148 degree 2 poles (-7.7169, 24.5406) (-7.6448, 24.5406) (-7.5216, 24.4944) (-7.4762, 24.4523) knots 0 0 0 1 2 2 2 construction
  spline S149 degree 2 poles (-7.4762, 24.4523) (-7.4309, 24.4101) (-7.3782, 24.2845) (-7.3782, 24.2067) knots 0 0 0 1 2 2 2 construction
  spline S150 degree 2 poles (-7.3782, 24.2067) (-7.3782, 24.1354) (-7.4098, 23.996) (-7.4349, 23.945) knots 0 0 0 1 2 2 2 construction
  line L147 (-7.4349, 23.945) -> (-7.5767, 23.945) construction
  line L148 (-7.5767, 23.945) -> (-7.5767, 23.9547) construction
  spline S151 degree 2 poles (-7.5767, 23.9547) (-7.5654, 23.9701) (-7.5362, 24.0276) (-7.5232, 24.0625) knots 0 0 0 1 2 2 2 construction
  spline S152 degree 2 poles (-7.5232, 24.0625) (-7.5095, 24.1022) (-7.4941, 24.1678) (-7.4941, 24.2092) knots 0 0 0 1 2 2 2 construction
  spline S153 degree 2 poles (-7.4941, 24.2092) (-7.4941, 24.2497) (-7.5232, 24.3259) (-7.5549, 24.3534) knots 0 0 0 1 2 2 2 construction
  spline S154 degree 2 poles (-7.5549, 24.3534) (-7.5848, 24.3785) (-7.6643, 24.4045) (-7.7177, 24.4045) knots 0 0 0 1 2 2 2 construction
  spline S155 degree 2 poles (-7.7177, 24.4045) (-7.7712, 24.4045) (-7.8393, 24.3753) (-7.862, 24.3477) knots 0 0 0 1 2 2 2 construction
  spline S156 degree 2 poles (-7.862, 24.3477) (-7.8871, 24.3194) (-7.9082, 24.2351) (-7.9082, 24.184) knots 0 0 0 1 2 2 2 construction
  spline S157 degree 2 poles (-7.9082, 24.184) (-7.9082, 24.1289) (-7.8912, 24.0195) (-7.8839, 23.9863) knots 0 0 0 1 2 2 2 construction
  spline S158 degree 2 poles (-8.422, 24.9871) (-8.422, 25.1233) (-8.2793, 25.2878) (-8.1675, 25.2878) knots 0 0 0 1 2 2 2 construction
  spline S159 degree 2 poles (-8.1675, 25.2878) (-8.1002, 25.2878) (-7.969, 25.2092) (-7.9317, 25.1354) knots 0 0 0 1 2 2 2 construction
  line L149 (-7.9317, 25.1354) -> (-7.9276, 25.1354) construction
  spline S160 degree 2 poles (-7.9276, 25.1354) (-7.8871, 25.2229) (-7.7704, 25.3129) (-7.678, 25.3129) knots 0 0 0 1 2 2 2 construction
  spline S161 degree 2 poles (-7.678, 25.3129) (-7.55, 25.3129) (-7.3766, 25.1265) (-7.3766, 24.9871) knots 0 0 0 1 2 2 2 construction
  spline S162 degree 2 poles (-7.3766, 24.9871) (-7.3766, 24.9126) (-7.4211, 24.7902) (-7.4625, 24.7472) knots 0 0 0 1 2 2 2 construction
  spline S163 degree 2 poles (-7.4625, 24.7472) (-7.503, 24.7051) (-7.6132, 24.6613) (-7.6756, 24.6613) knots 0 0 0 1 2 2 2 construction
  spline S164 degree 2 poles (-7.6756, 24.6613) (-7.7566, 24.6613) (-7.8928, 24.7481) (-7.9333, 24.8307) knots 0 0 0 1 2 2 2 construction
  line L150 (-7.9333, 24.8307) -> (-7.9373, 24.8307) construction
  spline S165 degree 2 poles (-7.9373, 24.8307) (-7.9803, 24.757) (-8.0824, 24.6857) (-8.1586, 24.6857) knots 0 0 0 1 2 2 2 construction
  spline S166 degree 2 poles (-8.1586, 24.6857) (-8.2712, 24.6857) (-8.422, 24.8558) (-8.422, 24.9871) knots 0 0 0 1 2 2 2 construction
  spline S167 degree 2 poles (-8.1675, 26.0382) (-8.1002, 26.0382) (-7.969, 25.9596) (-7.9317, 25.8858) knots 0 0 0 1 2 2 2 construction
  line L151 (-7.9317, 25.8858) -> (-7.9276, 25.8858) construction
  spline S168 degree 2 poles (-7.9276, 25.8858) (-7.8871, 25.9733) (-7.7704, 26.0633) (-7.678, 26.0633) knots 0 0 0 1 2 2 2 construction
  spline S169 degree 2 poles (-7.678, 26.0633) (-7.55, 26.0633) (-7.3766, 25.8769) (-7.3766, 25.7375) knots 0 0 0 1 2 2 2 construction
  spline S170 degree 2 poles (-7.3766, 25.7375) (-7.3766, 25.663) (-7.4211, 25.5406) (-7.4625, 25.4977) knots 0 0 0 1 2 2 2 construction
  spline S171 degree 2 poles (-7.4625, 25.4977) (-7.503, 25.4555) (-7.6132, 25.4118) (-7.6756, 25.4118) knots 0 0 0 1 2 2 2 construction
  spline S172 degree 2 poles (-7.6756, 25.4118) (-7.7566, 25.4118) (-7.8928, 25.4985) (-7.9333, 25.5811) knots 0 0 0 1 2 2 2 construction
  line L152 (-7.9333, 25.5811) -> (-7.9373, 25.5811) construction
  spline S173 degree 2 poles (-7.9373, 25.5811) (-7.9803, 25.5074) (-8.0824, 25.4361) (-8.1586, 25.4361) knots 0 0 0 1 2 2 2 construction
  spline S174 degree 2 poles (-8.1586, 25.4361) (-8.2712, 25.4361) (-8.422, 25.6062) (-8.422, 25.7375) knots 0 0 0 1 2 2 2 construction
  spline S175 degree 2 poles (-8.422, 25.7375) (-8.422, 25.8737) (-8.2793, 26.0382) (-8.1675, 26.0382) knots 0 0 0 1 2 2 2 construction
  line L153 (-7.4398, 26.1776) -> (-7.5816, 26.1776) construction
  line L154 (-7.5816, 26.1776) -> (-7.5816, 26.1873) construction
  spline S176 degree 2 poles (-7.5816, 26.1873) (-7.5508, 26.2294) (-7.4941, 26.372) (-7.4941, 26.4425) knots 0 0 0 1 2 2 2 construction
  spline S177 degree 2 poles (-7.4941, 26.4425) (-7.4941, 26.4839) (-7.52, 26.5665) (-7.55, 26.5941) knots 0 0 0 1 2 2 2 construction
  spline S178 degree 2 poles (-7.55, 26.5941) (-7.58, 26.6208) (-7.6513, 26.6492) (-7.7056, 26.6492) knots 0 0 0 1 2 2 2 construction
  spline S179 degree 2 poles (-7.7056, 26.6492) (-7.7599, 26.6492) (-7.8304, 26.6176) (-7.8506, 26.5892) knots 0 0 0 1 2 2 2 construction
  spline S180 degree 2 poles (-7.8506, 26.5892) (-7.8709, 26.5609) (-7.8863, 26.4839) (-7.8863, 26.4385) knots 0 0 0 1 2 2 2 construction
  line L155 (-7.8863, 26.4385) -> (-7.8863, 26.3818) construction
  line L156 (-7.8863, 26.3818) -> (-7.9973, 26.3818) construction
  line L157 (-7.9973, 26.3818) -> (-7.9973, 26.4263) construction
  spline S181 degree 2 poles (-7.9973, 26.4263) (-7.9973, 26.5163) (-8.0832, 26.6297) (-8.1651, 26.6297) knots 0 0 0 1 2 2 2 construction
  spline S182 degree 2 poles (-8.1651, 26.6297) (-8.2032, 26.6297) (-8.2574, 26.6006) (-8.2737, 26.5771) knots 0 0 0 1 2 2 2 construction
  spline S183 degree 2 poles (-8.2737, 26.5771) (-8.2907, 26.5519) (-8.3044, 26.4904) (-8.3044, 26.4555) knots 0 0 0 1 2 2 2 construction
  spline S184 degree 2 poles (-8.3044, 26.4555) (-8.3044, 26.419) (-8.2866, 26.3469) (-8.2728, 26.3121) knots 0 0 0 1 2 2 2 construction
  spline S185 degree 2 poles (-8.2728, 26.3121) (-8.2591, 26.2797) (-8.2299, 26.2318) (-8.2169, 26.2132) knots 0 0 0 1 2 2 2 construction
  line L158 (-8.2169, 26.2132) -> (-8.2169, 26.2051) construction
  line L159 (-8.2169, 26.2051) -> (-8.3587, 26.2051) construction
  spline S186 degree 2 poles (-8.3587, 26.2051) (-8.3822, 26.2489) (-8.4203, 26.3988) (-8.4203, 26.466) knots 0 0 0 1 2 2 2 construction
  spline S187 degree 2 poles (-8.4203, 26.466) (-8.4203, 26.5341) (-8.3928, 26.6354) (-8.3636, 26.6767) knots 0 0 0 1 2 2 2 construction
  spline S188 degree 2 poles (-8.3636, 26.6767) (-8.332, 26.7205) (-8.2404, 26.7659) (-8.1788, 26.7659) knots 0 0 0 1 2 2 2 construction
  spline S189 degree 2 poles (-8.1788, 26.7659) (-8.0962, 26.7659) (-7.9714, 26.6573) (-7.9552, 26.5811) knots 0 0 0 1 2 2 2 construction
  line L160 (-7.9552, 26.5811) -> (-7.9455, 26.5811) construction
  spline S190 degree 2 poles (-7.9455, 26.5811) (-7.939, 26.6127) (-7.9098, 26.6848) (-7.8806, 26.7156) knots 0 0 0 1 2 2 2 construction
  spline S191 degree 2 poles (-7.8806, 26.7156) (-7.8523, 26.7464) (-7.7615, 26.7853) (-7.6959, 26.7853) knots 0 0 0 1 2 2 2 construction
  spline S192 degree 2 poles (-7.6959, 26.7853) (-7.6286, 26.7853) (-7.5143, 26.7391) (-7.4706, 26.697) knots 0 0 0 1 2 2 2 construction
  spline S193 degree 2 poles (-7.4706, 26.697) (-7.4252, 26.6532) (-7.3782, 26.5293) (-7.3782, 26.4507) knots 0 0 0 1 2 2 2 construction
  spline S194 degree 2 poles (-7.3782, 26.4507) (-7.3782, 26.3753) (-7.4147, 26.2278) (-7.4398, 26.1776) knots 0 0 0 1 2 2 2 construction
  circle A0 centre (-15.045, 28.1037) radius 0.885 construction
  circle A1 centre (-15.045, 25.5637) radius 0.885 construction
  circle A2 centre (-15.045, 23.0237) radius 0.885 construction
  circle A3 centre (-15.045, 20.4837) radius 0.885 construction
  circle A4 centre (-15.045, 17.9437) radius 0.885 construction
  circle A5 centre (-15.045, 15.4037) radius 0.885 construction
  circle A6 centre (-15.045, 12.8637) radius 0.885 construction
  circle A7 centre (-15.045, 10.3237) radius 0.885 construction
  circle A8 centre (-2.465, 27.2837) radius 1.685 construction
  line L161 (0.2, 30.0687) -> (-16.92, 30.0687) construction
  line L162 (-16.92, 30.0687) -> (-16.92, 8.4487) construction
  line L163 (-16.92, 8.4487) -> (0.2, 8.4487) construction
  line L164 (0.2, 8.4487) -> (0.2, 30.0687) construction
  point P0 (-2.0533, 0)
  constraints: 1 coincident
hole "Hole1" at (-0.4117, 11.2609, -27.2837) direction (0, -1, 0) diameter 4 end through all countersink diameter 4.5 countersink angle 90
chamfer "Chamfer2" distance 0.8 angle 45 21 edges at (4.398, 2.9732, 0) (3.2931, 0.849, 0) (2.1882, -0.4084, 0) (3.2638, 5.1267, 0) (-6.3065, 6.2609, 0) (-15.8768, 5.1267, 0) (-17.011, 2.9732, 0) (-15.9061, 0.849, 0) (-15.3012, -1.0609, 0) (2.6882, -1.0609, 0) (3.2638, 5.1267, -45) (4.398, 2.9732, -45) (3.2931, 0.849, -45) (2.1882, -0.4084, -45) (-15.3012, -1.0609, -45) (-14.8012, -0.4084, -45) (-15.9061, 0.849, -45) (-17.011, 2.9732, -45) (-15.8768, 5.1267, -45) (-6.3065, 6.2609, -45) (2.6882, -1.0609, -45)
chamfer "Chamfer3" distance 0.2 angle 45 6 edges at (-15.0663, 12.5259, 0) (-14.8663, 13.2909, 0) (-14.8663, 11.7609, 0) (2.2533, 11.7609, 0) (2.4533, 12.5259, 0) (2.2533, 13.2909, 0)
equation "\"d5\" = d1"
body "Solid1"
